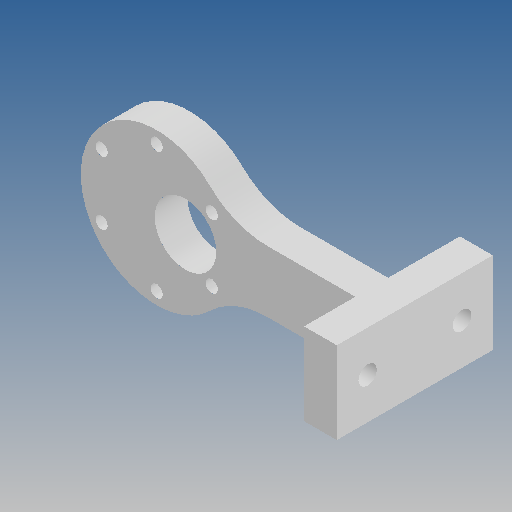
# Autodesk Inventor part: DCMotorHolder
Saved by Autodesk Inventor 2021 (Build 250183000, 183)
## iProperties
Created: 2022-09-08
Part Number: DCMotorHolder
Material: Generic
Document SubType Name: Modeling
Designer: Nathann
Density: 1 g/cm^3
Appearance: Default
Author: Nathann
Autodesk Inventor part; units mm, degrees
ref_plane "YZ Plane" through (0, 0, 0) normal (1, 0, 0) x (0, 1, 0)
ref_plane "XZ Plane" through (0, 0, 0) normal (0, 1, 0) x (-1, 0, 0)
ref_plane "XY Plane" through (0, 0, 0) normal (0, 0, 1) x (1, 0, 0)
sketch "Sketch1" plane through (0, 0, 0) normal (0, 0, 1) x (1, 0, 0)
  circle A0 centre (13.4234, -7.75) radius 1.5 projected
  circle A1 centre (-13.4234, -7.75) radius 1.5 projected
  circle A2 centre (0, 15.5) radius 1.5 projected
  circle A3 centre (-13.4234, 7.75) radius 1.5 projected
  circle A4 centre (0, -15.5) radius 1.5 projected
  circle A5 centre (13.4234, 7.75) radius 1.5 projected
  circle A6 centre (7, 0) radius 7 projected
  circle A7 centre (0, 0) radius 18.5 projected
  circle A8 centre (7, 0) radius 7.5
  line L0 (16.9115, 7.5) -> (51.9115, 7.5)
  line L1 (51.9115, 7.5) -> (51.9115, -7.5)
  line L2 (51.9115, -7.5) -> (16.9115, -7.5)
  line L3 (51.9115, -10) -> (58.9115, -10)
  line L4 (58.9115, -10) -> (58.9115, 10)
  line L5 (58.9115, 10) -> (51.9115, 10)
  line L6 (51.9115, 10) -> (51.9115, -10)
  point P0 (0, 0)
  point P1 (51.9115, -7.5)
  dimension "d0" = 15
  dimension "d1" = 35
  dimension "d2" = 20
  dimension "d3" = 7
  dimension "d4" = 2.5
  dimension "d5" = 0
  constraints: 14 end point, 3 perpendicular, 2 horizontal, 2 parallel, 2 point on circle, 1 centre point, 1 coincident, 1 horizontal alignment
  measures "d0" diameter of A8
  measures "d1" distance of L0.start L0.end
  measures "d2" distance of L3.end L4.end
  measures "d3" distance of L4.end L5.end
  measures "d4" distance between parallel lines of L0 L5
  measures "d5" distance between parallel lines of L1 L6
extrude "Extrusion1" add sketch "Sketch1" along normal blind 8 contours A7 | A7 L0 L1 L2 | L6 L5 L4 L3 L1
sketch "Sketch2" plane through (58.9115, -10, 0) normal (1, 0, 0) x (0, 0, -1)
  line L0 (-23, 20) -> (15, 20)
  line L1 (15, 20) -> (15, 0)
  line L2 (15, 0) -> (-23, 0)
  line L3 (-23, 0) -> (-23, 20)
  line L4 (0, 20) -> (-8, 20) projected
  line L5 (-8, 0) -> (-8, 20) projected
  circle A0 centre (7.5, 10) radius 2.25
  circle A1 centre (-15.5, 10) radius 2.25
  point P0 (0, 10)
  dimension "d8" = 20
  dimension "d9" = 0
  dimension "d10" = 38
  dimension "d11" = 15
  dimension "d12" = 4.5
  dimension "d13" = 4.5
  dimension "d14" = 7.5
  dimension "d15" = 7.5
  constraints: 8 end point, 2 centre point, 2 parallel, 1 horizontal, 1 perpendicular
  measures "d8" distance of L2.end L0.start
  measures "d9" distance between parallel lines of L0 L4
  measures "d10" distance of L0.start L0.end
  measures "d11" distance between parallel lines of L3 L5
  measures "d12" diameter of A0
  measures "d13" diameter of A1
  measures "d14" distance from line of L3 A1.centre
  measures "d15" distance from line of L1 A0.centre
extrude "Extrusion2" add sketch "Sketch2" against normal blind 8
fillet "Fillet1" radius 20 2 edges at (16.9115, 7.5, 4) (16.9115, -7.5, 4)
equation "\"d14\" = d15"
body "Solid1"
